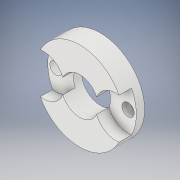
# Autodesk Inventor part: AA026
Saved by Autodesk Inventor 2017 SP1 (Build 210196100, 196)
## iProperties
Created: 2017-10-08
Part Number: AA026
Material: ABS Plastic
Document SubType Name: Modeling
Designer: Zach
Density: 1.06 g/cm^3
Appearance: CR White
Author: Zach
Autodesk Inventor part; units mm, degrees
ref_plane "YZ Plane" through (0, 0, 0) normal (1, 0, 0) x (0, 1, 0)
ref_plane "XZ Plane" through (0, 0, 0) normal (0, 1, 0) x (-1, 0, 0)
ref_plane "XY Plane" through (0, 0, 0) normal (0, 0, 1) x (1, 0, 0)
sketch "Sketch1" plane through (0, 0, 0) normal (0, 0, 1) x (1, 0, 0)
  circle A0 centre (0, 0) radius 10.75
  circle A1 centre (0, 0) radius 4.5
  line L0 (-8.75, 0) -> (8.75, 0) construction
  circle A2 centre (-8.75, 0) radius 1.5
  circle A3 centre (8.75, 0) radius 1.5
  dimension "d0" = 21.5
  dimension "d1" = 9
  dimension "d2" = 3
  dimension "d3" = 3
  dimension "d4" = 17.5
  constraints: 5 coincident, 4 centre point, 2 end point, 1 horizontal, 1 midpoint
  measures "d0" diameter of A0
  measures "d1" diameter of A1
  measures "d2" diameter of A2
  measures "d3" diameter of A3
  measures "d4" distance of L0.start L0.end
extrude "Extrusion1" add sketch "Sketch1" along normal blind 5
sketch "Sketch2" plane through (0, 0, 5) normal (0, 0, 1) x (1, 0, 0)
  circle A0 centre (-8.75, 0) radius 1.5 projected
  circle A1 centre (8.75, 0) radius 1.5 projected
  circle A2 centre (-8.75, 0) radius 5
  circle A3 centre (8.75, 0) radius 5
  point P0 (0, 0)
  dimension "d7" = 10
  dimension "d8" = 10
  constraints: 2 centre point, 2 coincident
  measures "d7" diameter of A2
  measures "d8" diameter of A3
extrude "Extrusion2" cut sketch "Sketch2" against normal blind 3
body "Solid1"
